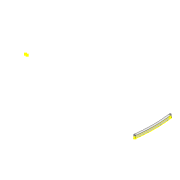
# Autodesk Inventor part: Part_4
Saved by Autodesk Inventor 2022 (Build 260153000, 153)
## iProperties
Created: 2022-04-26
Part Number: Part_4
Material: Generic
Document SubType Name: Modeling
Designer: dell
Density: 1 g/cm^3
Appearance: Default
Author: dell
Autodesk Inventor part; units mm, degrees
ref_plane "YZ Plane" through (0, 0, 0) normal (1, 0, 0) x (0, 1, 0)
ref_plane "XZ Plane" through (0, 0, 0) normal (0, 1, 0) x (-1, 0, 0)
ref_plane "XY Plane" through (0, 0, 0) normal (0, 0, 1) x (1, 0, 0)
sketch "Sketch1" plane through (0, 0, 0) normal (0, 1, 0) x (-1, 0, 0)
  line L0 (0, 0) -> (0, -111.226) construction
  line L1 (-3, 0) -> (-3, -111.226)
  line L2 (3, -111.226) -> (3, 0)
  arc A0 (3, 0) -> (-3, 0) centre (0, 0) ccw
  arc A1 (-3, -111.226) -> (3, -111.226) centre (0, -111.226) ccw
  circle A2 centre (0, 0) radius 1.5
  circle A3 centre (0, -111.226) radius 1.5
  arc A4 (3, 0) -> (3, -111.226) centre (399.1151, -55.613) ccw
  arc A5 (-3, 0) -> (-3, -111.226) centre (393.1151, -55.613) ccw
  point P0 (0, -55.613)
  dimension "d0" = 111.226
  dimension "d1" = 6
  dimension "d2" = 3
  dimension "d3" = 3
  dimension "d10" = 400
  dimension "d11" = 400
  constraints: 8 end point, 8 point on circle, 6 centre point, 4 tangent, 2 coincident, 1 midpoint, 1 parallel, 1 vertical
  measures "d0" distance of L0.start L0.end
  measures "d1" diameter of A1
  measures "d2" diameter of A2
  measures "d3" diameter of A3
  measures "d10" radius of A4
  measures "d11" radius of A5
extrude "Extrusion1" add sketch "Sketch1" along normal blind 8 contours A0 A4 A1 L1 | L1 A5
sketch "Sketch2" plane through (0, 0, 0) normal (0, -1, 0) x (1, 0, 0)
  arc A0 (3, 0) -> (-3, 0) centre (0, 0) ccw projected
  arc A1 (-3, -111.226) -> (-3, 0) centre (-399.1151, -55.613) ccw projected
  arc A2 (-3, -111.226) -> (3, -111.226) centre (0, -111.226) ccw projected
  arc A3 (3, -111.226) -> (3, 0) centre (-393.1151, -55.613) ccw projected
  circle A4 centre (0, -111.226) radius 1.5 projected
  circle A5 centre (0, 0) radius 1.5 projected
body "Solid1"
